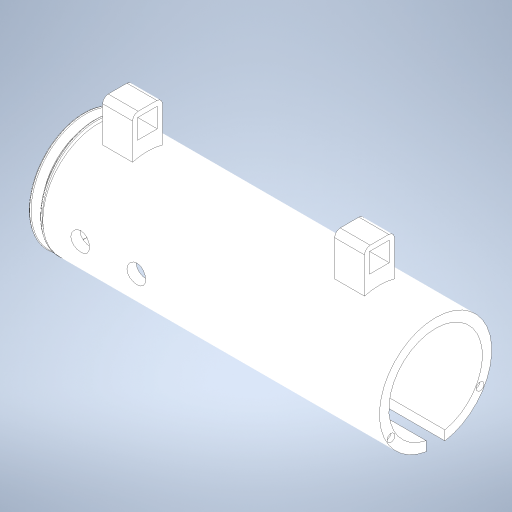
# Autodesk Inventor part: restrainer_middle
Saved by Autodesk Inventor 2023 (Build 270158000, 158)
## iProperties
Created: 2022-11-01
Part Number: restrainer_middle
Material: Generic
Document SubType Name: Modeling
Designer: Admin
Density: 1 g/cm^3
Appearance: Default
Author: Admin
Autodesk Inventor part; units mm, degrees
ref_plane "XZ Plane" through (0, 0, 0) normal (0, 1, 0) x (-1, 0, 0)
ref_plane "XY Plane" through (0, 0, 0) normal (0, 0, 1) x (1, 0, 0)
sketch "Sketch1" plane through (0, 0, 0) normal (1, 0, 0) x (0, 1, 0)
  circle A0 centre (0, 0) radius 15
  circle A1 centre (0, 0) radius 12.5
  circle A2 centre (-6.25, 0) radius 6.25
  line L0 (15, 0) -> (-15, 0)
  line L1 (-12.5, 0) -> (-12.5, 2.5)
  line L2 (-12.5, 0) -> (-12.5, -2.5)
  line L3 (-12.2474, -2.5) -> (-14.7902, -2.5)
  line L4 (-12.2474, 2.5) -> (-14.7902, 2.5)
  point P0 (-12.5, 0)
  dimension "d0" = 30
  dimension "d1" = 25
  dimension "d2" = 12.5
  dimension "d19" = 2.5
  dimension "d20" = 2.5
  constraints: 10 end point, 8 point on circle, 3 centre point, 2 coincident, 2 horizontal, 2 point on line, 2 tangent, 1 vertical
  measures "d0" diameter of A0
  measures "d1" diameter of A1
  measures "d2" diameter of A2
  measures "d19" distance of L1.start L1.end
  measures "d20" distance of L1.start L2.end
extrude "Extrusion1" add sketch "Sketch1" along normal blind 95 contours L0 A1 L4 A0 | A0 L3 A1 L0 | L4 L1 L0 A0 | A0 L0 L2 L3 | L4 A1 L1 | L2 A1 L3
extrude "Extrusion2" add sketch "Sketch1" along normal blind 2.5 contours L0 A2 A1 | A1 A2 L0
ref_plane "Work Plane1" through (10, 0, 0) normal (1, 0, 0) x (0, 1, 0)
sketch "Sketch5" plane through (10, 0, 0) normal (1, 0, 0) x (0, 1, 0)
  circle A0 centre (0, 0) radius 15
  circle A1 centre (0, 0) radius 12.5
  circle A2 centre (-6.25, 0) radius 6.25
  line L0 (15, 0) -> (-15, 0)
  line L1 (-12.5, 0) -> (-12.5, 2.5)
  line L2 (-12.5, 0) -> (-12.5, -2.5)
  line L3 (-12.2474, -2.5) -> (-14.7902, -2.5)
  line L4 (-12.2474, 2.5) -> (-14.7902, 2.5)
  line L5 (-11.9782, 2.5) -> (-12.5, 2.5)
  line L6 (-12.5, -2.5) -> (-11.9782, -2.5)
  point P0 (-12.5, 0)
  point P1 (-12.5, 0)
  point P2 (-12.5, 0)
  dimension "d22" = 30
  dimension "d23" = 25
  dimension "d24" = 12.5
  dimension "d25" = 2.5
  dimension "d26" = 2.5
  constraints: 14 end point, 10 point on circle, 3 centre point, 3 horizontal, 2 coincident, 2 point on line, 2 tangent, 1 collinear, 1 vertical
  measures "d22" diameter of A0
  measures "d23" diameter of A1
  measures "d24" diameter of A2
  measures "d25" distance of L1.start L1.end
  measures "d26" distance of L1.start L2.end
extrude "Extrusion4" cut sketch "Sketch5" along normal blind 110 contours L4 L1 L0 A0 | A0 L0 L2 L3 | L4 A1 L1 | L2 A1 L3
sketch "Sketch6" plane through (10, 0, 0) normal (1, 0, 0) x (0, 1, 0)
  line L0 (17.5, 4) -> (25.5, 4)
  line L1 (25.5, 4) -> (25.5, -4)
  line L2 (25.5, -4) -> (17.5, -4)
  line L3 (17.5, -4) -> (17.5, 4)
  line L4 (17.5, 4) -> (25.5, -4) construction
  line L5 (25.5, 4) -> (17.5, -4) construction
  line L6 (18.875, 2.625) -> (24.125, 2.625)
  line L7 (24.125, 2.625) -> (24.125, -2.625)
  line L8 (24.125, -2.625) -> (18.875, -2.625)
  line L9 (18.875, -2.625) -> (18.875, 2.625)
  line L10 (18.875, 2.625) -> (24.125, -2.625) construction
  line L11 (24.125, 2.625) -> (18.875, -2.625) construction
  line L12 (17.5, 0) -> (28.4919, 0)
  line L13 (17.5, -4) -> (16.9568, -4)
  line L14 (17.5, 4) -> (16.9568, 4)
  arc A0 (-14.7902, -2.5) -> (-14.7902, 2.5) centre (0, 0) ccw projected
  circle A1 centre (0, 0) radius 17.5
  line L15 (16.9568, 4) -> (14.4568, 4)
  line L16 (16.9568, -4) -> (14.4568, -4)
  point P0 (21.5, 0)
  dimension "d29" = 8
  dimension "d30" = 8
  dimension "d31" = 5.25
  dimension "d32" = 5.25
  dimension "d99" = 35
  constraints: 34 end point, 5 horizontal, 4 midpoint, 4 parallel, 2 perpendicular, 1 centre point, 1 coincident, 1 point on line, 1 tangent, 3 other
  measures "d29" distance of L1.end L2.end
  measures "d30" distance of L0.end L1.end
  measures "d31" distance of L7.end L8.end
  measures "d32" distance of L6.end L7.end
  measures "d99" diameter of A1
extrude "Extrusion5" add sketch "Sketch6" along normal blind 8 contours L0 L1 L12 L7 L6 L9 L3 | L3 A1 L14 | L12 L9 L8 L7 L1 L2 L3 | A1 L13 L16 A0 L15 L14 | L3 L13 A1 picked at (15.7929, 0)
pattern_linear "Rectangular Pattern2" count 2 spacing 62 along (1, 0, 0) of "Extrusion5"
fillet "Fillet2" radius 1.5 4 edges at (14, 25.5, 4) (14, 25.5, -4) (76, 25.5, -4) (76, 25.5, 4)
sketch "Sketch7" plane through (0, 0, 0) normal (0, 0, 1) x (1, 0, 0)
  circle A0 centre (15, 0) radius 2.5
  line L0 (0, -15) -> (0, 15) projected
  point P0 (0, 0)
  dimension "d39" = 5
  dimension "d42" = 15
  constraints: 1 centre point
  measures "d39" diameter of A0
  measures "d42" distance from line of L0 A0.centre
extrude "Extrusion6" cut sketch "Sketch7" along normal mid plane 50
pattern_linear "Rectangular Pattern3" count 2 spacing 15 along (1, 0, 0) of "Extrusion6"
sketch "Sketch14" plane through (95, 0, 0) normal (1, 0, 0) x (0, 0, -1)
  arc A0 (2.5, -14.7902) -> (-2.5, -14.7902) centre (0, 0) ccw projected
  arc A1 (2.5, -12.2474) -> (-2.5, -12.2474) centre (0, 0) ccw projected
  line L0 (0, 0) -> (0, 15)
  line L1 (0, 0) -> (-12.9904, -7.5)
  circle A2 centre (-11.9078, -6.875) radius 1.05
  arc A3 (-2.5, 25.5) -> (-4, 24) centre (-2.5, 24) ccw projected
  line L2 (-4, 24) -> (-4, 14.4568) projected
  arc A4 (4, 14.4568) -> (-4, 14.4568) centre (0, 0) ccw projected
  line L3 (4, 14.4568) -> (4, 24) projected
  arc A5 (4, 24) -> (2.5, 25.5) centre (2.5, 24) ccw projected
  line L4 (2.5, 25.5) -> (-2.5, 25.5) projected
  line L5 (2.625, 18.875) -> (-2.625, 18.875) projected
  line L6 (-2.625, 18.875) -> (-2.625, 24.125) projected
  line L7 (-2.625, 24.125) -> (2.625, 24.125) projected
  line L8 (2.625, 24.125) -> (2.625, 18.875) projected
  dimension "d94" = 120
  dimension "d95" = 2.1
  dimension "d96" = 0.2
  constraints: 4 end point, 2 point on circle, 1 centre point, 1 point on line
  measures "d94" angle of L0 L1
  measures "d95" diameter of A2
extrude "Extrusion7" cut sketch "Sketch14" against normal blind 1.1 contours A2 L1 | L1 A2
mirror "Mirror1" about plane through (0, 0, 0) normal (0, 0, 1) of "Extrusion7"
thread "Thread7" size "M30x3" class "6g" standard "ANSI Metric M Profile" length 5
sketch "Sketch22" plane through (0, 0, 0) normal (0, 1, 0) x (0, 0, 1)
  line L0 (15, 0) -> (15, 5)
  line L1 (15, 5) -> (12.7756, 5)
  line L2 (12.7756, 5) -> (12.7756, 0)
  line L3 (12.7756, 0) -> (15, 0)
  line L4 (0, -1) -> (0, 6) projected
  constraints: 8 end point
revolve "Revolution9" cut sketch "Sketch22" angle 360 about axis through (0, 0, 0) along (1, 0, 0)
sketch "Sketch23" plane through (0, 0, 0) normal (0, 1, 0) x (0, 0, 1)
  line L0 (15, 0) -> (15, 5)
  line L1 (15, 5) -> (12.7756, 5)
  line L2 (12.7756, 5) -> (12.7756, 0)
  line L3 (12.7756, 0) -> (15, 0)
  line L4 (0, -1) -> (0, 6) projected
  constraints: 8 end point
revolve "Revolution10" add sketch "Sketch23" angle 360 about axis through (0, 0, 0) along (1, 0, 0) separate body
sketch "Sketch21" plane through (0, 0, 0) normal (0, -1, 0) x (1, 0, 0)
  line L0 (-1.7501, -12.9275) -> (-1.5001, -12.9275) construction
  line L1 (0.2499, -14.8485) -> (-0.0001, -15.3287) construction
  line L2 (-3.0001, -15.3287) -> (-3.2501, -14.8485) construction
  line L3 (-1.2501, -12.9275) -> (-1.5001, -12.4472) construction
  line L4 (-1.5001, -12.4472) -> (-1.7501, -12.9275) construction
  line L5 (-3.0001, -15.3287) -> (-2.7501, -14.8485) construction
  line L6 (-1.2501, -12.9275) -> (-0.2501, -14.8485)
  line L7 (-3.2501, -14.8485) -> (-2.7501, -14.8485) construction
  arc A0 (-3.2501, -14.8485) -> (-3.0001, -15.0002) centre (-3.0001, -14.7183) ccw construction
  line L8 (0.2499, -14.8485) -> (-0.2501, -14.8485) construction
  line L9 (-3.0001, -15.3287) -> (-3.0001, -14.8485) construction
  line L10 (-0.0001, -15.3287) -> (-0.0001, -14.8485) construction
  line L11 (-1.5001, -12.4472) -> (-1.5001, -12.7758) construction
  line L12 (-3.0001, -15.0002) -> (-0.0001, -15.0002)
  arc A1 (-3.0001, -15.0002) -> (-2.7501, -14.8485) centre (-3.0001, -14.7183) ccw
  line L13 (-0.2501, -14.8485) -> (-0.0001, -15.3287) construction
  line L14 (-2.7501, -14.8485) -> (-1.7501, -12.9275)
  line L15 (-0.0001, -0.0002) -> (-0.0001, 0.0177)
  line L16 (-0.0001, 0.0177) -> (-0.0001, -0.0002)
  line L17 (-0.0001, -0.0002) -> (0.0334, -0.0002)
  arc A2 (-0.2501, -14.8485) -> (-0.0001, -15.0002) centre (-0.0001, -14.7183) ccw
  arc A3 (-0.0001, -15.0002) -> (0.2499, -14.8485) centre (-0.0001, -14.7183) ccw construction
  arc A4 (-1.5001, -12.7758) -> (-1.7501, -12.9275) centre (-1.5001, -13.0576) ccw
  arc A5 (-1.2501, -12.9275) -> (-1.5001, -12.7758) centre (-1.5001, -13.0576) ccw
  line L18 (-1.5001, -12.7758) -> (-1.5001, -12.9275) construction
  line L19 (-1.5001, -12.9275) -> (-1.2501, -12.9275) construction
  dimension "d144" = 55
  dimension "d145" = 0.4803
  dimension "d146" = 0.4803
  dimension "Sketch21_ThreadOffset" = 0
  dimension "Sketch21_MajorRadius" = 15
  dimension "d149" = 3
  dimension "Sketch21_MinorRadius" = 12.7756
  constraints: 40 end point, 12 point on circle, 10 parallel, 8 tangent, 6 centre point, 6 collinear, 2 midpoint, 2 point on line, 1 horizontal, 1 perpendicular, 3 other
  measures "d144" angle of L6 L14
  measures "d145" distance of L3.end L0.end
  measures "d146" distance of L1.end L10.end
  measures "Sketch21_ThreadOffset" distance between parallel lines of L15 L10
  measures "Sketch21_MajorRadius" distance from line of L12 L15.start
  measures "d149" distance from line of L1.end L9
  measures "Sketch21_MinorRadius" distance edge to line of A5 L17
coil "Coil5" sketch "Sketch21" operation cut axis through (0, 0, 0) along (1, 0, 0) pitch 3.003 turns 3.663004 hand right bodies 2
equation "\"d144\" = d151"
equation "\"d145\" = 0.160083 * Sketch21_Pitch"
equation "\"d146\" = 0.160083 * Sketch21_Pitch"
equation "\"d149\" = Sketch21_Pitch"
equation "\"d59\" = 55deg"
equation "\"Sketch8_Pitch\" = 3"
equation "\"d81\" = 55deg"
equation "\"Sketch11_Pitch\" = 2"
equation "\"d109\" = 55deg"
equation "\"Sketch15_Pitch\" = 2"
equation "\"d130\" = 55deg"
equation "\"Sketch18_Pitch\" = 2.5"
equation "\"d151\" = 55deg"
equation "\"Sketch21_Pitch\" = 3"
body "Solid1"
body "Solid6"
